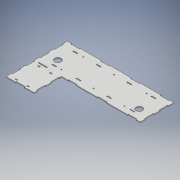
# Autodesk Inventor part: FLOOR-02
Saved by Autodesk Inventor 2018 (Build 220112000, 112)
## iProperties
Created: 2018-03-06
Part Number: FLOOR-02
Material: Generic
Document SubType Name: Modeling
Designer: isai
Density: 1 g/cm^3
Appearance: Default
Author: isai
Autodesk Inventor part; units mm, degrees
ref_plane "YZ Plane" through (0, 0, 0) normal (1, 0, 0) x (0, 1, 0)
sketch "Sketch1" plane through (0, 0, 0) normal (0, 0, 1) x (1, 0, 0)
  line L0 (29.5603, -99.2) -> (49.5603, -99.2)
  line L1 (49.5603, -103.2) -> (49.5603, -99.2)
  line L2 (29.5603, -103.2) -> (29.5603, -99.2)
  line L3 (70, -103.2) -> (70, -99.2)
  line L4 (73.6, -99.2) -> (73.6, -103.2)
  line L5 (25, 4) -> (25, 0)
  line L6 (45, 4) -> (45, 0)
  line L7 (70, 0) -> (70, 4)
  line L8 (73.6, 4) -> (73.6, 0)
  line L9 (134.1, 4) -> (134.1, 0)
  line L10 (154.1, 4) -> (154.1, 0)
  line L11 (214.6, 0) -> (214.6, 4)
  line L12 (218.2, 4) -> (218.2, 0)
  line L13 (277.1516, 4) -> (277.1516, 0)
  line L14 (297.1516, 4) -> (297.1516, 0)
  line L15 (366.4, 0) -> (366.4, 4)
  line L16 (370, 4) -> (370, 0)
  line L17 (390.4397, 4) -> (390.4397, 0)
  line L18 (410.4397, 4) -> (410.4397, 0)
  line L19 (395, -103.2) -> (395, -99.2)
  line L20 (415, -103.2) -> (415, -99.2)
  line L21 (370, -99.2) -> (370, -103.2)
  line L22 (366.4, -103.2) -> (366.4, -99.2)
  line L23 (305.9, -103.2) -> (305.9, -99.2)
  line L24 (285.9, -103.2) -> (285.9, -99.2)
  line L25 (221.8, -103.2) -> (221.8, -99.2)
  line L26 (225.4, -99.2) -> (225.4, -103.2)
  line L27 (162.8484, -103.2) -> (162.8484, -99.2)
  line L28 (142.8484, -103.2) -> (142.8484, -99.2)
  line L29 (25, 0) -> (45, 0)
  line L30 (70, 0) -> (73.6, 0)
  line L31 (134.1, 0) -> (154.1, 0)
  line L32 (214.6, 0) -> (218.2, 0)
  line L33 (277.1516, 0) -> (297.1516, 0)
  line L34 (366.4, 0) -> (370, 0)
  line L35 (390.4397, 0) -> (410.4397, 0)
  line L36 (49.5603, -103.2) -> (29.5603, -103.2)
  line L37 (70, -99.2) -> (73.6, -99.2)
  line L38 (70, -103.2) -> (73.6, -103.2)
  line L39 (142.8484, -99.2) -> (162.8484, -99.2)
  line L40 (142.8484, -103.2) -> (162.8484, -103.2)
  line L41 (221.8, -99.2) -> (225.4, -99.2)
  line L42 (221.8, -103.2) -> (225.4, -103.2)
  line L43 (285.9, -99.2) -> (305.9, -99.2)
  line L44 (285.9, -103.2) -> (305.9, -103.2)
  line L45 (366.4, -99.2) -> (370, -99.2)
  line L46 (366.4, -103.2) -> (370, -103.2)
  line L47 (395, -99.2) -> (415, -99.2)
  line L48 (395, -103.2) -> (415, -103.2)
  line L49 (469, 29) -> (469, -128.2)
  line L50 (469, -128.2) -> (49.5603, -128.2)
  line L51 (49.5603, -128.2) -> (-29, -128.2)
  line L52 (-29, -128.2) -> (-29, 29)
  line L53 (-29, 29) -> (469, 29)
  line L54 (25, 4) -> (45, 4)
  line L55 (70, 4) -> (73.6, 4)
  line L56 (70, -103.2) -> (73.6, -103.2)
  line L57 (142.8484, -103.2) -> (162.8484, -103.2)
  line L58 (221.8, -103.2) -> (225.4, -103.2)
  line L59 (285.9, -103.2) -> (305.9, -103.2)
  line L60 (366.4, -103.2) -> (370, -103.2)
  line L61 (395, -103.2) -> (415, -103.2)
  line L62 (390.4397, 4) -> (410.4397, 4)
  line L63 (366.4, 4) -> (370, 4)
  line L64 (277.1516, 4) -> (297.1516, 4)
  line L65 (134.1, 4) -> (154.1, 4)
  line L66 (214.6, 4) -> (218.2, 4)
  point P0 (0, 0)
  constraints: 134 end point, 11 parallel, 9 horizontal, 4 collinear, 3 perpendicular
extrude "Extrusion1" add sketch "Sketch1" along normal blind 4
sketch "Sketch2" plane through (0, 0, 0) normal (0, 0, -1) x (-1, 0, 0)
  line L0 (-162.8484, -99.2) -> (-142.8484, -99.2) projected
  line L1 (-142.8484, -99.2) -> (-142.8484, -103.2) projected
  line L2 (-142.8484, -103.2) -> (-162.8484, -103.2) projected
  line L3 (-162.8484, -103.2) -> (-162.8484, -99.2) projected
  line L4 (-154.1, 4) -> (-134.1, 4) projected
  line L5 (-134.1, 4) -> (-134.1, 0) projected
  line L6 (-134.1, 0) -> (-154.1, 0) projected
  line L7 (-154.1, 0) -> (-154.1, 4) projected
  line L8 (-285.9, -103.2) -> (-305.9, -103.2) projected
  line L9 (-305.9, -103.2) -> (-305.9, -99.2) projected
  line L10 (-305.9, -99.2) -> (-285.9, -99.2) projected
  line L11 (-285.9, -99.2) -> (-285.9, -103.2) projected
  line L12 (-297.1516, 4) -> (-277.1516, 4) projected
  line L13 (-277.1516, 4) -> (-277.1516, 0) projected
  line L14 (-277.1516, 0) -> (-297.1516, 0) projected
  line L15 (-297.1516, 0) -> (-297.1516, 4) projected
  line L16 (-395, -99.2) -> (-395, -103.2) projected
  line L17 (-395, -103.2) -> (-415, -103.2) projected
  line L18 (-415, -103.2) -> (-415, -99.2) projected
  line L19 (-415, -99.2) -> (-395, -99.2) projected
  line L20 (-410.4397, 4) -> (-390.4397, 4) projected
  line L21 (-390.4397, 4) -> (-390.4397, 0) projected
  line L22 (-390.4397, 0) -> (-410.4397, 0) projected
  line L23 (-410.4397, 0) -> (-410.4397, 4) projected
  line L24 (-25, 0) -> (-45, 0) projected
  line L25 (-45, 0) -> (-45, 4) projected
  line L26 (-45, 4) -> (-25, 4) projected
  line L27 (-25, 4) -> (-25, 0) projected
  line L28 (-49.5603, -103.2) -> (-49.5603, -99.2) projected
  line L29 (-49.5603, -99.2) -> (-29.5603, -99.2) projected
  line L30 (-29.5603, -99.2) -> (-29.5603, -103.2) projected
  line L31 (-29.5603, -103.2) -> (-49.5603, -103.2) projected
  line L32 (-221.8, -103.2) -> (-225.4, -103.2) projected
  line L33 (-225.4, -103.2) -> (-225.4, -99.2) projected
  line L34 (-225.4, -99.2) -> (-221.8, -99.2) projected
  line L35 (-221.8, -99.2) -> (-221.8, -103.2) projected
  line L36 (-370, -103.2) -> (-370, -99.2) projected
  line L37 (-370, -99.2) -> (-366.4, -99.2) projected
  line L38 (-366.4, -99.2) -> (-366.4, -103.2) projected
  line L39 (-366.4, -103.2) -> (-370, -103.2) projected
  line L40 (-218.2, 4) -> (-214.6, 4) projected
  line L41 (-214.6, 4) -> (-214.6, 0) projected
  line L42 (-214.6, 0) -> (-218.2, 0) projected
  line L43 (-218.2, 0) -> (-218.2, 4) projected
  line L44 (-370, 4) -> (-366.4, 4) projected
  line L45 (-366.4, 4) -> (-366.4, 0) projected
  line L46 (-366.4, 0) -> (-370, 0) projected
  line L47 (-370, 0) -> (-370, 4) projected
  line L48 (-70, 0) -> (-73.6, 0) projected
  line L49 (-73.6, 0) -> (-73.6, 4) projected
  line L50 (-73.6, 4) -> (-70, 4) projected
  line L51 (-70, 4) -> (-70, 0) projected
  line L52 (-73.6, -103.2) -> (-73.6, -99.2) projected
  line L53 (-73.6, -99.2) -> (-70, -99.2) projected
  line L54 (-70, -99.2) -> (-70, -103.2) projected
  line L55 (-70, -103.2) -> (-73.6, -103.2) projected
  line L56 (-469, 29) -> (-469, -128.2) projected
  line L57 (-469, -128.2) -> (29, -128.2) projected
  line L58 (29, -128.2) -> (29, 29) projected
  line L59 (29, 29) -> (-469, 29) projected
  line L60 (29, 29) -> (-469, 29) projected
  line L61 (9, 25) -> (-30.7, 25)
  line L62 (-30.7, 25) -> (-30.7, 29)
  line L63 (-30.7, 29) -> (9, 29)
  line L64 (9, 29) -> (9, 25)
  line L65 (-130.6333, 25) -> (-170.3333, 25)
  line L66 (-170.3333, 25) -> (-170.3333, 29)
  line L67 (-170.3333, 29) -> (-130.6333, 29)
  line L68 (-130.6333, 29) -> (-130.6333, 25)
  line L69 (-269.9667, 25) -> (-309.6667, 25)
  line L70 (-309.6667, 25) -> (-309.6667, 29)
  line L71 (-309.6667, 29) -> (-269.9667, 29)
  line L72 (-269.9667, 29) -> (-269.9667, 25)
  line L73 (-409.3, 25) -> (-449, 25)
  line L74 (-449, 25) -> (-449, 29)
  line L75 (-449, 29) -> (-409.3, 29)
  line L76 (-409.3, 29) -> (-409.3, 25)
  point P0 (0, 0)
  point P1 (9, 21)
  dimension "d3" = 39.7
  dimension "d4" = 4
  dimension "d5" = 39.7
  dimension "d6" = 4
  dimension "d7" = 39.7
  dimension "d8" = 39.7
  dimension "d9" = 4
  dimension "d10" = 20
  dimension "d11" = 20
  dimension "d12" = 378.6
  constraints: 32 end point, 8 parallel, 4 horizontal, 4 perpendicular, 1 point on line
  measures "d3" distance of L62.end L63.end
  measures "d4" distance of L61.end L62.end
  measures "d5" distance of L66.end L67.end
  measures "d6" distance of L65.end L66.end
  measures "d7" distance of L70.end L71.end
  measures "d8" distance of L74.end L75.end
  measures "d9" distance of L73.end L74.end
  measures "d10" distance between parallel lines of L64 L58
  measures "d11" distance from line of L56 L73.end
  measures "d12" distance of L75.end L62.end
extrude "Extrusion2" cut sketch "Sketch2" against normal blind 4 contours L59 L76 L73 L74 | L59 L72 L69 L70 | L64 L61 L62 L59 | L59 L68 L65 L66
ref_plane "Work Plane1" through (-29, -49.6, 0) normal (0, -1, 0) x (1, 0, 0)
mirror "Mirror1" about plane through (-29, -49.6, 0) normal (0, -1, 0) of "Extrusion2"
sketch "Sketch3" plane through (0, 0, 0) normal (0, 0, -1) x (-1, 0, 0)
  line L0 (-73.6, -103.2) -> (-73.6, -99.2) projected
  line L1 (-73.6, -99.2) -> (-70, -99.2) projected
  line L2 (-70, -99.2) -> (-70, -103.2) projected
  line L3 (-70, -103.2) -> (-73.6, -103.2) projected
  line L4 (-70, 0) -> (-73.6, 0) projected
  line L5 (-73.6, 0) -> (-73.6, 4) projected
  line L6 (-73.6, 4) -> (-70, 4) projected
  line L7 (-70, 4) -> (-70, 0) projected
  line L8 (-370, 4) -> (-366.4, 4) projected
  line L9 (-366.4, 4) -> (-366.4, 0) projected
  line L10 (-366.4, 0) -> (-370, 0) projected
  line L11 (-370, 0) -> (-370, 4) projected
  line L12 (-218.2, 4) -> (-214.6, 4) projected
  line L13 (-214.6, 4) -> (-214.6, 0) projected
  line L14 (-214.6, 0) -> (-218.2, 0) projected
  line L15 (-218.2, 0) -> (-218.2, 4) projected
  line L16 (-370, -103.2) -> (-370, -99.2) projected
  line L17 (-370, -99.2) -> (-366.4, -99.2) projected
  line L18 (-366.4, -99.2) -> (-366.4, -103.2) projected
  line L19 (-366.4, -103.2) -> (-370, -103.2) projected
  line L20 (-221.8, -103.2) -> (-225.4, -103.2) projected
  line L21 (-225.4, -103.2) -> (-225.4, -99.2) projected
  line L22 (-225.4, -99.2) -> (-221.8, -99.2) projected
  line L23 (-221.8, -99.2) -> (-221.8, -103.2) projected
  line L24 (-49.5603, -103.2) -> (-49.5603, -99.2) projected
  line L25 (-49.5603, -99.2) -> (-29.5603, -99.2) projected
  line L26 (-29.5603, -99.2) -> (-29.5603, -103.2) projected
  line L27 (-29.5603, -103.2) -> (-49.5603, -103.2) projected
  line L28 (-25, 0) -> (-45, 0) projected
  line L29 (-45, 0) -> (-45, 4) projected
  line L30 (-45, 4) -> (-25, 4) projected
  line L31 (-25, 4) -> (-25, 0) projected
  line L32 (-410.4397, 4) -> (-390.4397, 4) projected
  line L33 (-390.4397, 4) -> (-390.4397, 0) projected
  line L34 (-390.4397, 0) -> (-410.4397, 0) projected
  line L35 (-410.4397, 0) -> (-410.4397, 4) projected
  line L36 (-395, -99.2) -> (-395, -103.2) projected
  line L37 (-395, -103.2) -> (-415, -103.2) projected
  line L38 (-415, -103.2) -> (-415, -99.2) projected
  line L39 (-415, -99.2) -> (-395, -99.2) projected
  line L40 (-297.1516, 4) -> (-277.1516, 4) projected
  line L41 (-277.1516, 4) -> (-277.1516, 0) projected
  line L42 (-277.1516, 0) -> (-297.1516, 0) projected
  line L43 (-297.1516, 0) -> (-297.1516, 4) projected
  line L44 (-285.9, -103.2) -> (-305.9, -103.2) projected
  line L45 (-305.9, -103.2) -> (-305.9, -99.2) projected
  line L46 (-305.9, -99.2) -> (-285.9, -99.2) projected
  line L47 (-285.9, -99.2) -> (-285.9, -103.2) projected
  line L48 (-154.1, 4) -> (-134.1, 4) projected
  line L49 (-134.1, 4) -> (-134.1, 0) projected
  line L50 (-134.1, 0) -> (-154.1, 0) projected
  line L51 (-154.1, 0) -> (-154.1, 4) projected
  line L52 (-162.8484, -99.2) -> (-142.8484, -99.2) projected
  line L53 (-142.8484, -99.2) -> (-142.8484, -103.2) projected
  line L54 (-142.8484, -103.2) -> (-162.8484, -103.2) projected
  line L55 (-162.8484, -103.2) -> (-162.8484, -99.2) projected
  line L56 (-309.6667, -128.2) -> (-309.6667, -124.2) projected
  line L57 (-309.6667, -124.2) -> (-269.9667, -124.2) projected
  line L58 (-269.9667, -124.2) -> (-269.9667, -128.2) projected
  line L59 (-269.9667, -128.2) -> (-170.3333, -128.2) projected
  line L60 (-170.3333, -128.2) -> (-170.3333, -124.2) projected
  line L61 (-170.3333, -124.2) -> (-130.6333, -124.2) projected
  line L62 (-130.6333, -124.2) -> (-130.6333, -128.2) projected
  line L63 (-130.6333, -128.2) -> (-30.7, -128.2) projected
  line L64 (-30.7, -128.2) -> (-30.7, -124.2) projected
  line L65 (-30.7, -124.2) -> (9, -124.2) projected
  line L66 (9, -124.2) -> (9, -128.2) projected
  line L67 (9, -128.2) -> (29, -128.2) projected
  line L68 (29, -128.2) -> (29, 29) projected
  line L69 (29, 29) -> (9, 29) projected
  line L70 (9, 29) -> (9, 25) projected
  line L71 (9, 25) -> (-30.7, 25) projected
  line L72 (-30.7, 25) -> (-30.7, 29) projected
  line L73 (-30.7, 29) -> (-130.6333, 29) projected
  line L74 (-130.6333, 29) -> (-130.6333, 25) projected
  line L75 (-130.6333, 25) -> (-170.3333, 25) projected
  line L76 (-170.3333, 25) -> (-170.3333, 29) projected
  line L77 (-170.3333, 29) -> (-269.9667, 29) projected
  line L78 (-269.9667, 29) -> (-269.9667, 25) projected
  line L79 (-269.9667, 25) -> (-309.6667, 25) projected
  line L80 (-309.6667, 25) -> (-309.6667, 29) projected
  line L81 (-309.6667, 29) -> (-409.3, 29) projected
  line L82 (-409.3, 29) -> (-409.3, 25) projected
  line L83 (-409.3, 25) -> (-449, 25) projected
  line L84 (-449, 25) -> (-449, 29) projected
  line L85 (-449, 29) -> (-469, 29) projected
  line L86 (-469, 29) -> (-469, -128.2) projected
  line L87 (-469, -128.2) -> (-449, -128.2) projected
  line L88 (-449, -128.2) -> (-449, -124.2) projected
  line L89 (-449, -124.2) -> (-409.3, -124.2) projected
  line L90 (-409.3, -124.2) -> (-409.3, -128.2) projected
  line L91 (-409.3, -128.2) -> (-309.6667, -128.2) projected
  line L92 (29, 29) -> (29, -128.2) projected
  line L93 (29, -103.2) -> (25, -103.2)
  line L94 (25, -103.2) -> (25, -63.5)
  line L95 (25, -63.5) -> (29, -63.5)
  line L96 (29, -63.5) -> (29, -103.2)
  line L97 (29, -35.7) -> (25, -35.7)
  line L98 (25, -35.7) -> (25, 4)
  line L99 (25, 4) -> (29, 4)
  line L100 (29, 4) -> (29, -35.7)
  point P0 (0, 0)
  dimension "d18" = 39.7
  dimension "d19" = 4
  dimension "d20" = 39.7
  dimension "d21" = 4
  dimension "d22" = 157.2
  constraints: 16 end point, 4 parallel, 2 horizontal, 2 perpendicular, 2 point on line
  measures "d18" distance of L93.end L94.end
  measures "d19" distance of L98.end L99.end
  measures "d20" distance of L97.end L98.end
  measures "d21" distance of L93.start L93.end
  measures "d22" distance between parallel lines of L69 L67
extrude "Extrusion3" cut sketch "Sketch3" against normal blind 4 contours L93 L94 L95 L68 | L97 L98 L99 L68
ref_plane "Work Plane2" through (220, -128.2, 0) normal (1, 0, 0) x (0, 0, -1)
mirror "Mirror2" about plane through (220, -128.2, 0) normal (1, 0, 0) of "Extrusion3"
sketch "Sketch7" plane through (0, 0, 0) normal (0, 0, -1) x (-1, 0, 0)
  line L0 (29, -128.2) -> (-101, -128.2)
  line L1 (-101, -128.2) -> (-101, -258.2)
  line L2 (-101, -258.2) -> (29, -258.2)
  line L3 (29, -258.2) -> (29, -128.2)
  point P0 (0, 0)
  dimension "d31" = 130
  dimension "d32" = 130
  constraints: 8 end point, 2 parallel, 1 horizontal, 1 perpendicular
  measures "d31" distance of L2.end L1.end
  measures "d32" distance of L1.end L0.end
extrude "Extrusion5" add sketch "Sketch7" against normal blind 4
sketch "Sketch8" plane through (0, 0, 0) normal (0, 0, -1) x (-1, 0, 0)
  line L0 (-30.7, -128.2) -> (-30.7, -124.2) projected
  line L1 (-30.7, -124.2) -> (9, -124.2) projected
  line L2 (9, -124.2) -> (9, -128.2) projected
  line L3 (9, -128.2) -> (-30.7, -128.2) projected
  line L4 (-101, -128.2) -> (-101, -258.2) projected
  line L5 (-101, -258.2) -> (29, -258.2) projected
  line L6 (29, -258.2) -> (29, -103.2) projected
  line L7 (29, -103.2) -> (25, -103.2) projected
  line L8 (25, -103.2) -> (25, -63.5) projected
  line L9 (25, -63.5) -> (29, -63.5) projected
  line L10 (29, -63.5) -> (29, -35.7) projected
  line L11 (29, -35.7) -> (25, -35.7) projected
  line L12 (25, -35.7) -> (25, 4) projected
  line L13 (25, 4) -> (29, 4) projected
  line L14 (29, 4) -> (29, 29) projected
  line L15 (29, 29) -> (9, 29) projected
  line L16 (9, 29) -> (9, 25) projected
  line L17 (9, 25) -> (-30.7, 25) projected
  line L18 (-30.7, 25) -> (-30.7, 29) projected
  line L19 (-30.7, 29) -> (-130.6333, 29) projected
  line L20 (-130.6333, 29) -> (-130.6333, 25) projected
  line L21 (-130.6333, 25) -> (-170.3333, 25) projected
  line L22 (-170.3333, 25) -> (-170.3333, 29) projected
  line L23 (-170.3333, 29) -> (-269.9667, 29) projected
  line L24 (-269.9667, 29) -> (-269.9667, 25) projected
  line L25 (-269.9667, 25) -> (-309.6667, 25) projected
  line L26 (-309.6667, 25) -> (-309.6667, 29) projected
  line L27 (-309.6667, 29) -> (-409.3, 29) projected
  line L28 (-409.3, 29) -> (-409.3, 25) projected
  line L29 (-409.3, 25) -> (-449, 25) projected
  line L30 (-449, 25) -> (-449, 29) projected
  line L31 (-449, 29) -> (-469, 29) projected
  line L32 (-469, 29) -> (-469, 4) projected
  line L33 (-469, 4) -> (-465, 4) projected
  line L34 (-465, 4) -> (-465, -35.7) projected
  line L35 (-465, -35.7) -> (-469, -35.7) projected
  line L36 (-469, -35.7) -> (-469, -63.5) projected
  line L37 (-469, -63.5) -> (-465, -63.5) projected
  line L38 (-465, -63.5) -> (-465, -103.2) projected
  line L39 (-465, -103.2) -> (-469, -103.2) projected
  line L40 (-469, -103.2) -> (-469, -128.2) projected
  line L41 (-469, -128.2) -> (-449, -128.2) projected
  line L42 (-449, -128.2) -> (-449, -124.2) projected
  line L43 (-449, -124.2) -> (-409.3, -124.2) projected
  line L44 (-409.3, -124.2) -> (-409.3, -128.2) projected
  line L45 (-409.3, -128.2) -> (-309.6667, -128.2) projected
  line L46 (-309.6667, -128.2) -> (-309.6667, -124.2) projected
  line L47 (-309.6667, -124.2) -> (-269.9667, -124.2) projected
  line L48 (-269.9667, -124.2) -> (-269.9667, -128.2) projected
  line L49 (-269.9667, -128.2) -> (-170.3333, -128.2) projected
  line L50 (-170.3333, -128.2) -> (-170.3333, -124.2) projected
  line L51 (-170.3333, -124.2) -> (-130.6333, -124.2) projected
  line L52 (-130.6333, -124.2) -> (-130.6333, -128.2) projected
  line L53 (-130.6333, -128.2) -> (-101, -128.2) projected
  line L54 (-162.8484, -99.2) -> (-142.8484, -99.2) projected
  line L55 (-142.8484, -99.2) -> (-142.8484, -103.2) projected
  line L56 (-142.8484, -103.2) -> (-162.8484, -103.2) projected
  line L57 (-162.8484, -103.2) -> (-162.8484, -99.2) projected
  line L58 (-154.1, 4) -> (-134.1, 4) projected
  line L59 (-134.1, 4) -> (-134.1, 0) projected
  line L60 (-134.1, 0) -> (-154.1, 0) projected
  line L61 (-154.1, 0) -> (-154.1, 4) projected
  line L62 (-285.9, -103.2) -> (-305.9, -103.2) projected
  line L63 (-305.9, -103.2) -> (-305.9, -99.2) projected
  line L64 (-305.9, -99.2) -> (-285.9, -99.2) projected
  line L65 (-285.9, -99.2) -> (-285.9, -103.2) projected
  line L66 (-297.1516, 4) -> (-277.1516, 4) projected
  line L67 (-277.1516, 4) -> (-277.1516, 0) projected
  line L68 (-277.1516, 0) -> (-297.1516, 0) projected
  line L69 (-297.1516, 0) -> (-297.1516, 4) projected
  line L70 (-395, -99.2) -> (-395, -103.2) projected
  line L71 (-395, -103.2) -> (-415, -103.2) projected
  line L72 (-415, -103.2) -> (-415, -99.2) projected
  line L73 (-415, -99.2) -> (-395, -99.2) projected
  line L74 (-410.4397, 4) -> (-390.4397, 4) projected
  line L75 (-390.4397, 4) -> (-390.4397, 0) projected
  line L76 (-390.4397, 0) -> (-410.4397, 0) projected
  line L77 (-410.4397, 0) -> (-410.4397, 4) projected
  line L78 (-25, 0) -> (-45, 0) projected
  line L79 (-45, 0) -> (-45, 4) projected
  line L80 (-45, 4) -> (-25, 4) projected
  line L81 (-25, 4) -> (-25, 0) projected
  line L82 (-49.5603, -103.2) -> (-49.5603, -99.2) projected
  line L83 (-49.5603, -99.2) -> (-29.5603, -99.2) projected
  line L84 (-29.5603, -99.2) -> (-29.5603, -103.2) projected
  line L85 (-29.5603, -103.2) -> (-49.5603, -103.2) projected
  line L86 (-221.8, -103.2) -> (-225.4, -103.2) projected
  line L87 (-225.4, -103.2) -> (-225.4, -99.2) projected
  line L88 (-225.4, -99.2) -> (-221.8, -99.2) projected
  line L89 (-221.8, -99.2) -> (-221.8, -103.2) projected
  line L90 (-370, -103.2) -> (-370, -99.2) projected
  line L91 (-370, -99.2) -> (-366.4, -99.2) projected
  line L92 (-366.4, -99.2) -> (-366.4, -103.2) projected
  line L93 (-366.4, -103.2) -> (-370, -103.2) projected
  line L94 (-218.2, 4) -> (-214.6, 4) projected
  line L95 (-214.6, 4) -> (-214.6, 0) projected
  line L96 (-214.6, 0) -> (-218.2, 0) projected
  line L97 (-218.2, 0) -> (-218.2, 4) projected
  line L98 (-370, 4) -> (-366.4, 4) projected
  line L99 (-366.4, 4) -> (-366.4, 0) projected
  line L100 (-366.4, 0) -> (-370, 0) projected
  line L101 (-370, 0) -> (-370, 4) projected
  line L102 (-70, 0) -> (-73.6, 0) projected
  line L103 (-73.6, 0) -> (-73.6, 4) projected
  line L104 (-73.6, 4) -> (-70, 4) projected
  line L105 (-70, 4) -> (-70, 0) projected
  line L106 (-73.6, -103.2) -> (-73.6, -99.2) projected
  line L107 (-73.6, -99.2) -> (-70, -99.2) projected
  line L108 (-70, -99.2) -> (-70, -103.2) projected
  line L109 (-70, -103.2) -> (-73.6, -103.2) projected
  line L110 (29, -103.2) -> (29, -258.2) projected
  line L111 (29, -233.2) -> (25, -233.2)
  line L112 (25, -233.2) -> (25, -193.5)
  line L113 (25, -193.5) -> (29, -193.5)
  line L114 (29, -193.5) -> (29, -233.2)
  line L115 (29, -128.5) -> (25, -128.5)
  line L116 (25, -128.5) -> (25, -168.2)
  line L117 (25, -168.2) -> (29, -168.2)
  line L118 (29, -168.2) -> (29, -128.5)
  line L119 (-101, -136.2372) -> (-97, -136.2372)
  line L120 (-97, -136.2372) -> (-97, -175.9372)
  line L121 (-97, -175.9372) -> (-101, -175.9372)
  line L122 (-101, -175.9372) -> (-101, -136.2372)
  line L123 (-101, -258.2) -> (-101, -128.2) projected
  line L124 (-101, -201.139) -> (-97, -201.139)
  line L125 (-97, -201.139) -> (-97, -240.839)
  line L126 (-97, -240.839) -> (-101, -240.839)
  line L127 (-101, -240.839) -> (-101, -201.139)
  line L128 (-16.15, -254.2) -> (-55.85, -254.2)
  line L129 (-55.85, -254.2) -> (-55.85, -258.2)
  line L130 (-55.85, -258.2) -> (-16.15, -258.2)
  line L131 (-16.15, -258.2) -> (-16.15, -254.2)
  point P0 (0, 0)
  point P1 (-36, -258.2)
  dimension "d35" = 4
  dimension "d36" = 39.7
  dimension "d37" = 25
  dimension "d38" = 4
  dimension "d39" = 39.7
  dimension "d51" = 4
  dimension "d52" = 39.7
  dimension "d53" = 4
  dimension "d54" = 39.7
  dimension "d55" = 39.7
  dimension "d56" = 4
  constraints: 40 end point, 10 parallel, 5 horizontal, 5 perpendicular, 4 point on line, 2 midpoint
  measures "d35" distance of L112.end L113.end
  measures "d36" distance of L111.end L112.end
  measures "d37" distance between parallel lines of L111 L5
  measures "d38" distance of L117.end L116.end
  measures "d39" distance of L116.end L115.end
  measures "d51" distance of L120.end L121.end
  measures "d52" distance of L119.end L120.end
  measures "d53" distance of L125.end L126.end
  measures "d54" distance of L124.end L125.end
  measures "d55" distance of L130.end L129.end
  measures "d56" distance of L129.end L128.end
extrude "Extrusion6" cut sketch "Sketch8" against normal blind 4 contours L111 L112 L113 L6 | L117 L116 L115 L6
extrude "Extrusion7" cut sketch "Sketch8" against normal blind 4 contours L119 L120 L121 L4 | L124 L125 L126 L4 | L129 L128 L131 L5
sketch "Sketch10" plane through (0, 0, 0) normal (0, 0, -1) x (-1, 0, 0)
  circle A0 centre (-414, -78.2) radius 15
  line L0 (-409.3, -128.2) -> (-309.6667, -128.2) projected
  line L1 (-469, -103.2) -> (-469, -128.2) projected
  circle A1 centre (-26, -71) radius 15
  line L2 (-30.7, 29) -> (-130.6333, 29) projected
  line L3 (29, -63.5) -> (29, -35.7) projected
  point P0 (0, 0)
  dimension "d59" = 30
  dimension "d60" = 50
  dimension "d61" = 55
  dimension "d62" = 30
  dimension "d63" = 100
  dimension "d64" = 55
  constraints: 2 centre point
  measures "d59" diameter of A0
  measures "d60" distance from line of L0 A0.centre
  measures "d61" distance from line of L1 A0.centre
  measures "d62" diameter of A1
  measures "d63" distance from line of A1.centre L2
  measures "d64" distance from line of A1.centre L3
extrude "Extrusion8" cut sketch "Sketch10" against normal blind 4
sketch "Sketch11" plane through (0, 0, 0) normal (0, 0, -1) x (-1, 0, 0)
  line L0 (-12, -138.3) -> (-2, -138.3)
  line L1 (-57, -248.3) -> (-67, -248.3)
  line L2 (-67, -244.3) -> (-57, -244.3)
  line L3 (-2, -248.3) -> (-12, -248.3)
  line L4 (-12, -244.3) -> (-2, -244.3)
  line L5 (-12, -248.3) -> (-12, -244.3)
  line L6 (-2, -248.3) -> (-2, -244.3)
  line L7 (-57, -248.3) -> (-57, -244.3)
  line L8 (-67, -248.3) -> (-67, -244.3)
  line L9 (-57, -142.3) -> (-67, -142.3)
  line L10 (-67, -138.3) -> (-57, -138.3)
  line L11 (-67, -138.3) -> (-67, -142.3)
  line L12 (-57, -138.3) -> (-57, -142.3)
  line L13 (-2, -142.3) -> (-12, -142.3)
  line L14 (-12, -138.3) -> (-12, -142.3)
  line L15 (-2, -138.3) -> (-2, -142.3)
  line L16 (-81, -248.3) -> (12, -248.3)
  line L17 (12, -248.3) -> (12, -138.3)
  line L18 (12, -138.3) -> (-81, -138.3)
  line L19 (-81, -138.3) -> (-81, -248.3)
  line L20 (-101, -240.839) -> (-101, -258.2) projected
  line L21 (-101, -258.2) -> (25, -258.2)
  line L22 (25, -258.2) -> (25, -128.5)
  line L23 (25, -128.5) -> (-101, -128.5)
  line L24 (-101, -128.5) -> (-101, -258.2)
  line L25 (29, -35.7) -> (29, -63.5) projected
  point P0 (0, 0)
  point P1 (-38, -193.3)
  point P2 (29, -193.3)
  constraints: 48 end point, 4 parallel, 2 horizontal, 2 perpendicular, 1 point on line
extrude "Extrusion9" cut sketch "Sketch11" against normal blind 10 contours L0 L15 L13 L14 | L12 L9 L11 L10 | L3 L5 L4 L6 | L8 L2 L7 L1
equation "\"d3\" = D"
equation "\"d5\" = D"
equation "\"d7\" = D"
equation "\"d8\" = D"
equation "\"d18\" = D"
equation "\"d20\" = D"
equation "\"d36\" = D"
equation "\"d39\" = D"
equation "\"d52\" = D"
equation "\"d54\" = D"
equation "\"d55\" = D"
equation "\"D\" = 39.7"
body "Solid1"
